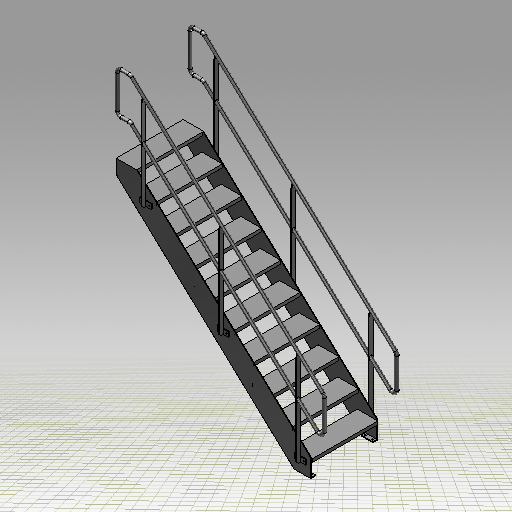
# Autodesk Inventor part: Stairs
Saved by Autodesk Inventor 2026.2 (Build 302298000, 298)
## iProperties
Created: 2015-02-12
Part Number: Stairs
Material: Steel
Document SubType Name: Modeling
Designer: Marc
Density: 7.85 g/cm^3
Appearance: Steel Galvanized
Mass: 1.1558e+06 g
Surface Area: 180796 cm^2
Volume: 147236 cm^3
Author: Marc
Autodesk Inventor part; units mm, degrees
sketch "MotherSketch" plane through (0, 0, 0) normal (0, 1, 0) x (-1, 0, 0)
  line L0 (0, 0) -> (0, 221)
  line L1 (0, 221) -> (2122.2177, 2200)
  line L2 (2122.2177, 2200) -> (2372.2177, 2200)
  line L3 (2122.2177, 2200) -> (2122.2177, 2160)
  line L4 (2122.2177, 2160) -> (2372.2177, 2160)
  line L5 (2372.2177, 2160) -> (2372.2177, 2200)
  line L6 (0, 221) -> (-236.9935, 0)
  line L7 (-236.9935, 0) -> (0, 0) construction
  line L8 (1935.2242, 1879) -> (2075.2242, 1879)
  line L9 (2075.2242, 1879) -> (2075.2242, 1939)
  line L10 (2075.2242, 1939) -> (1935.2242, 1939)
  line L11 (1935.2242, 1939) -> (1935.2242, 1879)
  line L12 (2075.2242, 1909) -> (2050.2242, 1909) construction
  line L13 (2050.2242, 1909) -> (1960.2242, 1909) construction
  line L14 (1960.2242, 1909) -> (1935.2242, 1909) construction
  circle A0 centre (2050.2242, 1909) radius 9
  circle A1 centre (1960.2242, 1909) radius 9
  line L15 (2000.2242, 1879) -> (2010.2242, 1879)
  line L16 (2010.2242, 1879) -> (2010.2242, 3056.4048)
  line L17 (2010.2242, 3056.4048) -> (2000.2242, 3056.4048)
  line L18 (2000.2242, 3056.4048) -> (2000.2242, 1879)
  line L19 (2322.2177, 3152) -> (2322.2177, 2748)
  line L20 (2274.2177, 2700) -> (2178.1189, 2700)
  line L21 (2145.3829, 2687.105) -> (-119.2641, 575.2875)
  line L22 (-200, 610.3924) -> (-200, 979.129)
  line L23 (-184.7359, 1014.234) -> (2145.3829, 3187.105)
  line L24 (2178.1189, 3200) -> (2274.2177, 3200)
  arc A2 (2178.1189, 3200) -> (2145.3829, 3187.105) centre (2178.1189, 3152) ccw
  arc A3 (2322.2177, 3152) -> (2274.2177, 3200) centre (2274.2177, 3152) ccw
  arc A4 (2274.2177, 2700) -> (2322.2177, 2748) centre (2274.2177, 2748) ccw
  arc A5 (2178.1189, 2700) -> (2145.3829, 2687.105) centre (2178.1189, 2652) ccw
  arc A6 (-200, 610.3924) -> (-119.2641, 575.2875) centre (-152, 610.3924) ccw
  arc A7 (-184.7359, 1014.234) -> (-200, 979.129) centre (-152, 979.129) ccw
  line L25 (2372.2177, 2160) -> (2372.2177, 2022.9305)
  line L26 (2372.2177, 2022.9305) -> (202.8903, 0)
  line L27 (202.8903, 0) -> (0, 0)
  line L28 (2122.2177, 2160) -> (1885.2242, 1939) construction
  line L29 (1885.2242, 1939) -> (1935.2242, 1939) construction
  point P0 (2005.2242, 1879)
  point P1 (2322.2177, 3200)
  point P2 (2322.2177, 2700)
  point P3 (-200, 500)
  point P4 (-200, 1000)
  point P5 (2005.2242, 3056.4048)
  dimension "StepHeight" = 221
  dimension "StepLenght" = 250
  dimension "StairsHeight" = 2200
  dimension "StairsAngle" = 43
  dimension "StepThickness" = 40
  dimension "StairsHypo" = 3225.8142
  dimension "StepHypo" = 324.0477
  dimension "d7" = 140
  dimension "d8" = 60
  dimension "d9" = 18
  dimension "d10" = 18
  dimension "d11" = 90
  dimension "d12" = 10
  dimension "d13" = 1000
  dimension "d14" = 500
  dimension "d15" = 500
  dimension "d19" = 1000
  dimension "d20" = 48
  dimension "d22" = 50
  dimension "d25" = 200
  dimension "d26" = 300
  dimension "d36" = 324.0477
  dimension "d37" = 50
  constraints: 60 end point, 12 point on circle, 12 tangent, 11 parallel, 11 perpendicular, 9 point on line, 8 centre point, 5 equal radius, 5 midpoint, 3 collinear, 2 coincident, 2 horizontal, 1 vertical
  measures "StepHeight" distance of L0.start L0.end
  measures "StepLenght" distance of L1.end L2.end
  measures "StairsHeight" distance from line of L0.start L2
  measures "StairsAngle" angle of L1 L2
  measures "StepThickness" distance of L1.end L3.end
  measures "StairsHypo" distance of L6.end L1.end
  measures "StepHypo" distance of L0.end L6.end
  measures "d7" distance of L10.end L9.end
  measures "d8" distance of L9.end L8.end
  measures "d9" diameter of A0
  measures "d10" diameter of A1
  measures "d11" distance of L12.end L13.end
  measures "d12" distance of L16.end L17.end
  measures "d13" distance between parallel lines of L2 L24
  measures "d14" distance of point (2322.218, 3200) point (2322.218, 2700)
  measures "d15" distance of point (-200, 500) point (-200, 1000)
  measures "d19" vertical distance of L0.start point (-200, 1000)
  measures "d20" radius of A2
  measures "d22" distance between parallel lines of L19 L5
  measures "d25" distance between parallel lines of L0 L22
  measures "d26" distance between parallel lines of L26 L1
  measures "d36" distance of L3.end L28.end
  measures "d37" distance of L28.end L10.end
extrude "UpperStep" add sketch "MotherSketch" along normal mid plane 800 contours L4 L3 L2 L5
pattern_linear "Steps Pattern" count 10 spacing 324.0477 along (0.7314, 0, -0.682) of "UpperStep"
sketch "Sketch2" plane through (0, -400, 0) normal (0, -1, 0) x (1, 0, 0)
  line L0 (-2122.2177, 2160) -> (-2122.2177, 2200) projected
  line L1 (-2122.2177, 2200) -> (-2372.2177, 2200) projected
  line L2 (-2372.2177, 2200) -> (-2372.2177, 2160) projected
  line L3 (-2372.2177, 2160) -> (-2122.2177, 2160) projected
  line L4 (0, 221) -> (-2122.2177, 2200) projected
  line L5 (-2372.2177, 2022.9305) -> (-202.8903, 0) projected
  line L6 (-2372.2177, 2160) -> (-2372.2177, 2022.9305) projected
  line L7 (0, 0) -> (0, 221) projected
  line L8 (-202.8903, 0) -> (0, 0) projected
extrude "LeftSidePlate" add sketch "Sketch2" along normal blind 8
sketch "Sketch3" plane through (0, -408, 0) normal (0, -1, 0) x (1, 0, 0)
  line L0 (-2075.2242, 1939) -> (-1935.2242, 1939) projected
  line L1 (-2075.2242, 1879) -> (-2075.2242, 1939) projected
  line L2 (-1935.2242, 1879) -> (-2075.2242, 1879) projected
  line L3 (-1935.2242, 1939) -> (-1935.2242, 1879) projected
  circle A0 centre (-1960.2242, 1909) radius 9 projected
  circle A1 centre (-2050.2242, 1909) radius 9 projected
extrude "LeftSideSpilConnectionPlate" add sketch "Sketch3" along normal blind 10
sketch "Sketch4" plane through (0, -418, 0) normal (0, -1, 0) x (1, 0, 0)
  line L0 (-2000.2242, 3056.4048) -> (-2000.2242, 1879) projected
  line L1 (-2010.2242, 1879) -> (-2010.2242, 3056.4048) projected
  line L2 (-2000.2242, 1879) -> (-2010.2242, 1879) projected
  line L3 (-2010.2242, 3056.4048) -> (-2000.2242, 3056.4048) projected
  point P0 (0, 0)
  point P1 (-2262.6483, 1903.5455)
  point P2 (-2272.6483, 1903.5455)
  constraints: 3 other
extrude "LeftSideSpil" add sketch "Sketch4" along normal blind 50
chamfer "LeftSideSpilChamfer1" distance 25 angle 45 1 edges at (-2005.2242, -468, 1879)
chamfer "LeftSideSpilChamfer2" distance 60 distance2 20 1 edges at (-2005.2242, -468, 3056.4048) measured on face at (-2006.8909, -468, 2672.2699)
chamfer "LeftSideSpilChamfer3" distance 60 distance2 20 1 edges at (-2005.2242, -418, 3056.4048) measured on face at (-2006.8909, -418, 2683.9366)
ref_plane "LeftRailingCenter" through (-2000.2242, -443, 3056.4048) normal (0, -1, 0) x (1, 0, 0)
sketch "Sketch5" plane through (-2000.2242, -443, 3056.4048) normal (0, -1, 0) x (1, 0, 0)
  line L0 (2184.9601, -2042.1708) -> (-145.1588, 130.7002) projected
  arc A0 (-145.1588, 130.7002) -> (-177.8947, 143.5952) centre (-177.8947, 95.5952) ccw projected
  line L1 (-177.8947, 143.5952) -> (-273.9935, 143.5952) projected
  arc A1 (-273.9935, 143.5952) -> (-321.9935, 95.5952) centre (-273.9935, 95.5952) ccw projected
  line L2 (-321.9935, 95.5952) -> (-321.9935, -308.4048) projected
  arc A2 (-321.9935, -308.4048) -> (-273.9935, -356.4048) centre (-273.9935, -308.4048) ccw projected
  line L3 (-273.9935, -356.4048) -> (-177.8947, -356.4048) projected
  arc A3 (-145.1588, -369.2998) -> (-177.8947, -356.4048) centre (-177.8947, -404.4048) ccw projected
  line L4 (-145.1588, -369.2998) -> (2119.4883, -2481.1174) projected
  arc A4 (2119.4883, -2481.1174) -> (2200.2242, -2446.0124) centre (2152.2242, -2446.0124) ccw projected
  line L5 (2200.2242, -2446.0124) -> (2200.2242, -2077.2758) projected
  arc A5 (2200.2242, -2077.2758) -> (2184.9601, -2042.1708) centre (2152.2242, -2077.2758) ccw projected
  point P0 (2000.2242, -3056.4048)
ref_plane "Work Plane2" through (-2178.1189, -443, 3200) normal (-1, 0, 0) x (0, -1, 0)
sketch "Sketch6" plane through (-2178.1189, -443, 3200) normal (-1, 0, 0) x (0, -1, 0)
  circle A0 centre (0, 0) radius 21.2
  circle A1 centre (0, 0) radius 18
  point P0 (-443, -3200)
  dimension "d51" = 42.4
  dimension "d126" = 3.2
  constraints: 2 centre point, 1 coincident
  measures "d51" diameter of A0
  measures "d126" radial gap between concentric circles of A0 A1
pattern_linear "LeftSideSpilPattern" count 3 spacing 1288.8594 along (0.7314, 0, -0.682) of "LeftSideSpilConnectionPlate", "LeftSideSpil", "LeftSideSpilChamfer1", "LeftSideSpilChamfer2", "LeftSideSpilChamfer3"
sketch "Sketch12" plane through (0, -400, 0) normal (0, 1, 0) x (1, 0, 0)
  line L0 (-2372.2177, -2160) -> (-2362.2177, -2160)
  line L1 (-2362.2177, -2160) -> (-2362.2177, -2020)
  line L2 (-2362.2177, -2020) -> (-2372.2177, -2020)
  line L3 (-2372.2177, -2020) -> (-2372.2177, -2160)
  dimension "d78" = 10
  dimension "d79" = 140
  constraints: 8 end point, 2 parallel, 1 horizontal, 1 perpendicular
  measures "d78" distance of L2.end L1.end
  measures "d79" distance of L1.end L0.end
extrude "Extrusion9" add sketch "Sketch12" along normal blind 50
sketch "Sketch13" plane through (-2362.2177, -400, 2160) normal (1, 0, 0) x (0, 0, -1)
  line L0 (140, 0) -> (140, 50) projected
  line L1 (0, 0) -> (0, 50) projected
  line L2 (0, 25) -> (25, 25)
  line L3 (25, 25) -> (115, 25)
  line L4 (115, 25) -> (140, 25)
  point P0 (2160, 400)
  dimension "d82" = 90
  constraints: 6 end point, 2 collinear, 2 midpoint, 1 perpendicular
  measures "d82" distance of L2.end L3.end
hole "Hole1" at (-2362.2177, -375, 2135) at (-2362.2177, -375, 2045) direction (-1, 0, 0) diameter 18 end through all
sketch "Sketch7" plane through (0, 400, 0) normal (0, 1, 0) x (1, 0, 0)
  line L0 (-2122.2177, -2200) -> (-2122.2177, -2160) projected
  line L1 (-2122.2177, -2160) -> (-2372.2177, -2160) projected
  line L2 (0, -221) -> (-2122.2177, -2200) projected
  line L3 (-2372.2177, -2022.9305) -> (-202.8903, 0) projected
  line L4 (-2372.2177, -2160) -> (-2372.2177, -2022.9305) projected
  line L5 (-202.8903, 0) -> (0, 0) projected
  line L6 (0, 0) -> (0, -221) projected
  line L7 (-2122.2177, -2200) -> (-2122.2177, -2160) projected
  line L8 (-2122.2177, -2160) -> (-2372.2177, -2160) projected
  line L9 (-2372.2177, -2160) -> (-2372.2177, -2200) projected
  line L10 (-2372.2177, -2200) -> (-2122.2177, -2200) projected
extrude "RightSidePlate" add sketch "Sketch7" along normal blind 8
sketch "Sketch8" plane through (0, 408, 0) normal (0, 1, 0) x (1, 0, 0)
  line L0 (-2075.2242, -1939) -> (-1935.2242, -1939) projected
  line L1 (-2075.2242, -1879) -> (-2075.2242, -1939) projected
  line L2 (-1935.2242, -1879) -> (-2075.2242, -1879) projected
  line L3 (-1935.2242, -1939) -> (-1935.2242, -1879) projected
  circle A0 centre (-1960.2242, -1909) radius 9 projected
  circle A1 centre (-2050.2242, -1909) radius 9 projected
extrude "RightSideSpilConnectionPlate" add sketch "Sketch8" along normal blind 10
sketch "Sketch9" plane through (0, 418, 0) normal (0, 1, 0) x (1, 0, 0)
  line L0 (-2000.2242, -3056.4048) -> (-2000.2242, -1879) projected
  line L1 (-2010.2242, -1879) -> (-2010.2242, -3056.4048) projected
  line L2 (-2000.2242, -1879) -> (-2010.2242, -1879) projected
  line L3 (-2010.2242, -3056.4048) -> (-2000.2242, -3056.4048) projected
  point P0 (0, 0)
extrude "RightSideSpil" add sketch "Sketch9" along normal blind 50
chamfer "RightSideChamfer4" distance 60 distance2 20 1 edges at (-2005.2242, 468, 3056.4048) measured on face at (-2003.5575, 468, 2663.9366)
chamfer "RightSideChamfer5" distance 60 distance2 20 1 edges at (-2005.2242, 418, 3056.4048) measured on face at (-2003.5575, 418, 2683.9366)
chamfer "RightSideChamfer6" distance 25 angle 45 1 edges at (-2005.2242, 468, 1879)
ref_plane "Work Plane3" through (-2000.2242, 443, 3056.4048) normal (0, 1, 0) x (-1, 0, 0)
sketch "Sketch10" plane through (-2000.2242, 443, 3056.4048) normal (0, 1, 0) x (-1, 0, 0)
  line L0 (177.8947, 143.5952) -> (273.9935, 143.5952) projected
  arc A0 (177.8947, 143.5952) -> (145.1588, 130.7002) centre (177.8947, 95.5952) ccw projected
  arc A1 (321.9935, 95.5952) -> (273.9935, 143.5952) centre (273.9935, 95.5952) ccw projected
  line L1 (321.9935, 95.5952) -> (321.9935, -308.4048) projected
  arc A2 (273.9935, -356.4048) -> (321.9935, -308.4048) centre (273.9935, -308.4048) ccw projected
  line L2 (273.9935, -356.4048) -> (177.8947, -356.4048) projected
  arc A3 (177.8947, -356.4048) -> (145.1588, -369.2998) centre (177.8947, -404.4048) ccw projected
  line L3 (145.1588, -369.2998) -> (-2119.4883, -2481.1174) projected
  line L4 (-2184.9601, -2042.1708) -> (145.1588, 130.7002) projected
  arc A4 (-2200.2242, -2446.0124) -> (-2119.4883, -2481.1174) centre (-2152.2242, -2446.0124) ccw projected
  line L5 (-2200.2242, -2446.0124) -> (-2200.2242, -2077.2758) projected
  arc A5 (-2184.9601, -2042.1708) -> (-2200.2242, -2077.2758) centre (-2152.2242, -2077.2758) ccw projected
  point P0 (-2000.2242, -3056.4048)
ref_plane "Work Plane4" through (-2178.1189, 443, 3200) normal (-1, 0, 0) x (0, -1, 0)
sketch "Sketch11" plane through (-2178.1189, 443, 3200) normal (-1, 0, 0) x (0, -1, 0)
  circle A0 centre (0, 0) radius 21.2
  circle A1 centre (0, 0) radius 18
  point P0 (443, -3200)
  dimension "d73" = 42.4
  dimension "d128" = 3.2
  constraints: 2 centre point, 1 coincident
  measures "d73" diameter of A0
  measures "d128" radial gap between concentric circles of A0 A1
pattern_linear "RightSideSpilPattern" count 3 spacing 1288.8594 along (0.7314, 0, -0.682) of "RightSideSpilConnectionPlate", "RightSideSpil", "RightSideChamfer4", "RightSideChamfer5", "RightSideChamfer6"
sketch "Sketch14" plane through (0, 400, 0) normal (0, -1, 0) x (1, 0, 0)
  line L0 (-2372.2177, 2160) -> (-2362.2177, 2160)
  line L1 (-2362.2177, 2160) -> (-2362.2177, 2020)
  line L2 (-2362.2177, 2020) -> (-2372.2177, 2020)
  line L3 (-2372.2177, 2020) -> (-2372.2177, 2160)
  dimension "d90" = 10
  dimension "d91" = 140
  constraints: 8 end point, 2 parallel, 1 horizontal, 1 perpendicular
  measures "d90" distance of L1.end L2.end
  measures "d91" distance of L0.end L1.end
extrude "Extrusion10" add sketch "Sketch14" along normal blind 50
sketch "Sketch15" plane through (-2362.2177, 400, 2160) normal (1, 0, 0) x (0, 0, -1)
  line L0 (0, -50) -> (0, 0) projected
  line L1 (140, 0) -> (140, -50) projected
  line L2 (0, -25) -> (25, -25)
  line L3 (25, -25) -> (115, -25)
  line L4 (115, -25) -> (140, -25)
  point P0 (2160, -400)
  dimension "d94" = 90
  constraints: 6 end point, 2 collinear, 2 midpoint, 1 perpendicular
  measures "d94" distance of L2.end L3.end
hole "Hole2" at (-2362.2177, 375, 2135) at (-2362.2177, 375, 2045) direction (-1, 0, 0) diameter 18 end through all
sketch "Sketch16" plane through (0, -400, 0) normal (0, 1, 0) x (1, 0, 0)
  line L0 (0, 0) -> (-140, 0)
  line L1 (-140, 0) -> (-140, -10)
  line L2 (-140, -10) -> (0, -10)
  line L3 (0, -10) -> (0, 0)
  dimension "d102" = 140
  dimension "d103" = 10
  constraints: 8 end point, 2 parallel, 1 horizontal, 1 perpendicular
  measures "d102" distance of L2.end L1.end
  measures "d103" distance of L1.end L0.end
extrude "Extrusion11" add sketch "Sketch16" along normal blind 50
sketch "Sketch17" plane through (-140, -400, 10) normal (0, 0, 1) x (1, 0, 0)
  line L0 (140, 0) -> (140, 50) projected
  line L1 (0, 0) -> (0, 50) projected
  line L2 (140, 25) -> (115, 25)
  line L3 (115, 25) -> (25, 25)
  line L4 (25, 25) -> (0, 25)
  point P0 (140, 400)
  dimension "d106" = 90
  constraints: 6 end point, 2 collinear, 2 midpoint, 1 perpendicular
  measures "d106" distance of L2.end L3.end
hole "Hole3" at (-115, -375, 10) at (-25, -375, 10) direction (0, 0, -1) diameter 18 end through all
sketch "Sketch18" plane through (0, 400, 0) normal (0, -1, 0) x (1, 0, 0)
  line L0 (0, 0) -> (-140, 0)
  line L1 (-140, 0) -> (-140, 10)
  line L2 (-140, 10) -> (0, 10)
  line L3 (0, 10) -> (0, 0)
  dimension "d114" = 140
  dimension "d115" = 10
  constraints: 8 end point, 2 parallel, 1 horizontal, 1 perpendicular
  measures "d114" distance of L1.end L2.end
  measures "d115" distance of L0.end L1.end
extrude "Extrusion12" add sketch "Sketch18" along normal blind 50
sketch "Sketch19" plane through (-140, 400, 10) normal (0, 0, 1) x (1, 0, 0)
  line L0 (0, 0) -> (0, -50) projected
  line L1 (140, 0) -> (140, -50) projected
  line L2 (0, -25) -> (25, -25)
  line L3 (25, -25) -> (115, -25)
  line L4 (115, -25) -> (140, -25)
  point P0 (140, -400)
  dimension "d118" = 90
  constraints: 6 end point, 2 collinear, 2 midpoint, 1 perpendicular
  measures "d118" distance of L2.end L3.end
hole "Hole4" at (-115, 375, 10) at (-25, 375, 10) direction (0, 0, -1) diameter 18 end through all
sweep "Sweep3" add profiles "Sketch6" path "Sketch5"
sweep "Sweep4" add profiles "Sketch11" path "Sketch10"
equation "\"d36\" = StepHypo"
equation "\"d35\" = StepHypo"
equation "\"d42\" = 0.5 * Spilthickness"
equation "\"d80\" = Spilthickness"
equation "\"d58\" = SidePlateThicknes"
equation "\"d60\" = SpliConnectionplateThickness"
equation "\"d62\" = Spilthickness"
equation "\"d70\" = 0.5 * Spilthickness"
equation "\"d92\" = Spilthickness"
equation "\"d104\" = Spilthickness"
equation "\"Spilthickness\" = 50"
equation "\"SidePlateThicknes\" = 8"
equation "\"SpliConnectionplateThickness\" = 10"
body "Solid1"
